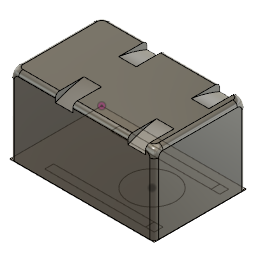
DAWA 6.1-MLX (Autodesk Fusion 360 design; units mm, degrees)
Autodesk Fusion 360 part; units mm, degrees
note: some values were not read from the file. Set by a fixed rule: which face or edge a step refers to.
sketch "Sketch1" plane through (0, 0, 0) normal (0, 1, 0) x (1, 0, 0)
  line L0 (0, 0) -> (33, 0)
  line L1 (33, 0) -> (33, -21)
  line L2 (33, -21) -> (0, -21)
  line L3 (0, -21) -> (0, 0)
  circle A0 centre (22, -10.5) radius 5.35
  line L4 (6, -2) -> (6, -4)
  line L5 (6, -4) -> (31, -4)
  line L6 (31, -4) -> (31, -2)
  line L7 (31, -2) -> (6, -2)
  line L8 (6, -19) -> (6, -17)
  line L9 (6, -17) -> (31, -17)
  line L10 (6, -19) -> (31, -19)
  line L11 (31, -19) -> (31, -17)
  line L12 (29, -2) -> (29, -4)
  line L13 (29, -17) -> (29, -19)
  dimension "d1" = 33
  dimension "d2" = 21
  dimension "d3" = 10.7
  dimension "d4" = 11
  dimension "d5" = 10.5
  dimension "d11" = 6
  dimension "d13" = 2
  dimension "d14" = 2
  dimension "d17" = 2
  dimension "d18" = 2
  dimension "d19" = 2
  dimension "d20" = 2
  dimension "d21" = 2
  constraint horizontal L0
  constraint vertical L1
  constraint horizontal L2
  constraint vertical L3
  constraint coincident L0.start L3.end
  constraint perpendicular L0 L4
  constraint perpendicular L4 L5
  constraint perpendicular L5 L6
  constraint perpendicular L6 L7
  constraint perpendicular L2 L8
  constraint perpendicular L8 L9
  constraint perpendicular L8 L10
  constraint perpendicular L9 L11
  constraint collinear L4 L8
  constraint coincident L7 L12.start
  constraint coincident L5 L12.end
  constraint perpendicular L5 L12
  constraint coincident L9 L13.start
  constraint coincident L10 L13.end
  constraint perpendicular L10 L13
  constraint collinear L12 L13
  measures "d1" distance of L0.start L0.end
  measures "d2" distance of L0.end L1.end
  measures "d3" diameter of A0
  measures "d4" distance of L1 A0.centre
  measures "d5" distance of L2 A0.centre
  measures "d11" distance of L3 L4
  measures "d13" distance of L5.end L6.end
  measures "d14" distance of L9.end L10.end
  measures "d17" distance of L2 L10
  measures "d18" distance of L1 L11
  measures "d19" distance of L1 L6
  measures "d20" distance of L0 L7
  measures "d21" distance of L6 L12
extrude "Extrude1" add sketch "Sketch1" along normal blind 18.2 contours L0 L1 L2 L3 | A0 | L4 L5 L7 L12 | L5 L6 L7 L12 | L8 L9 L10 L13 | L9 L10 L11 L13
shell "Shell1" thickness 2 removed faces 1 at (0, 6.0667, 14)
extrude "Extrude2" add 1 faces at (10.3333, 16.2, 7.6667) along direction (0, -1, 0) blind 1
extrude "Extrude3" add sketch "Sketch1" along normal blind 6 from surface at 2 contours L4 L5 L7 L12 | L8 L9 L10 L13
extrude "Extrude4" add sketch "Sketch1" along normal up to surface (13.2 mm away) from surface at 2 contours L5 L6 L7 L12 | L9 L10 L11 L13
extrude "Extrude5" cut sketch "Sketch1" along normal blind 3 contours A0
fillet "Fillet1" radius 0.5 2 edges at (17.012, 2, 8.5654) (17.012, 0, 12.4346)
sketch "Sketch2" plane through (0, 0, 0) normal (1, 0, 0) x (0, 0, -1)
  line L0 (-10.5, -8) -> (20, -8)
  line L1 (-10.5, -8) -> (-41, -8)
  arc A0 (20, -8) -> (-41, -8) centre (-10.5, -8) ccw
  arc A1 (16, -8) -> (-37, -8) centre (-10.5, -8) ccw
  constraint horizontal L0
  constraint parallel L0 L1
  constraint coincident L0.start L1.start
  constraint coincident L1 A1.end
  constraint coincident L0 A1.start
fillet "Fillet2" radius 1 8 edges at (16.5, 18.2, 21) (33, 18.2, 10.5) (16.5, 18.2, 0) (33, 9.1, 21) (0, 9.1, 21) (0, 9.1, 0) (33, 9.1, 0) (0, 18.2, 10.5)
extrude "Extrude6" cut sketch "Sketch2" against normal blind 4 from surface at 31 contours L0 L1 A0 A1
extrude "Extrude7" cut sketch "Sketch2" against normal blind 4 from surface at 14.4 contours L0 L1 A0 A1
named bodies: "Main"
